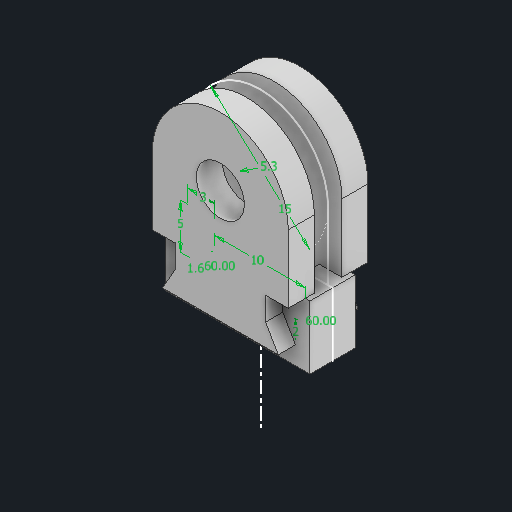
# Autodesk Inventor part: base
Saved by Autodesk Inventor 2026.2 (Build 302298000, 298)
## iProperties
Created: 2025-11-24
Part Number: base
Material: 一般
Document SubType Name: Modeling
Designer: 陳泓任
Density: 1 g/cm^3
Appearance: 預設
Author: 陳泓任
Autodesk Inventor part; units mm, degrees
ref_plane "YZ Plane" through (0, 0, 0) normal (1, 0, 0) x (0, 1, 0)
ref_plane "XZ Plane" through (0, 0, 0) normal (0, 1, 0) x (-1, 0, 0)
ref_plane "XY Plane" through (0, 0, 0) normal (0, 0, 1) x (1, 0, 0)
sketch "草圖1" plane through (0, 0, 0) normal (0, 0, 1) x (1, 0, 0)
  line L0 (0, 14.1483) -> (0, -10.3645)
  line L1 (0, 0) -> (-8, 0)
  line L2 (-8, 0) -> (-8, 7)
  line L3 (-8, 7) -> (-5, 7)
  line L4 (0, 0) -> (8, 0)
  line L5 (8, 0) -> (8, 7)
  line L6 (8, 7) -> (5, 7)
  circle A0 centre (0, 14.5) radius 2.65
  circle A1 centre (0, 14.5) radius 7.5 construction
  line L7 (-5, 4.4249) -> (-6.4, 2)
  line L8 (-6.4, 2) -> (0.3304, 2)
  line L9 (0.3304, 2) -> (6.4, 2)
  line L10 (6.4, 2) -> (5, 4.4249)
  line L11 (5, 4.4249) -> (5, 7)
  arc A2 (7.5, 14.5) -> (-7.5, 14.5) centre (0, 14.5) ccw
  line L12 (-7.5, 14.5) -> (-7.5, 7)
  line L13 (7.5, 14.5) -> (7.5, 7)
  line L14 (-5, 4.4249) -> (-5, 7)
  line L15 (-5, 4.4249) -> (5, 4.4249)
  point P0 (0, 2)
  dimension "d5" = 3
  dimension "d7" = 5.3
  dimension "d14" = 15
  dimension "d19" = 60
  dimension "d20" = 1.6
  dimension "d21" = 2
  dimension "d22" = 60
  dimension "d23" = 10
  dimension "d24" = 5
  constraints: 32 end point, 4 horizontal, 4 perpendicular, 4 point on circle, 4 point on line, 4 vertical, 3 centre point, 3 symmetric about line, 3 tangent, 1 coincident, 1 concentric
  measures "d5" distance of L3.end L2.end
  measures "d7" diameter of A0
  measures "d14" diameter of A1
  measures "d19" angle of L8 L7
  measures "d20" distance from line of L2 L7.end
  measures "d21" distance between parallel lines of L4 L9
  measures "d22" angle of L9 L10
  measures "d23" distance of L7.start L10.end
  measures "d24" distance between parallel lines of L8 L3
extrude "擠出1" add sketch "草圖1" along normal mid plane 5 contours L8 L9 L10 L11 L6 L5 L4 L0 | L0 L1 L2 L3 L14 L7 L8
extrude "擠出2" add sketch "草圖1" along normal mid plane 8.8 separate body contours L15 L14 L3 L12 A2 L13 L6 L11 | L15 L10 L9 L8 L0 | L0 L8 L7 L15
extrude "擠出3" cut sketch "草圖1" along normal mid plane 3.05 contours L15 L14 L3 L12 A2 L13 L6 L11 bodies 2
